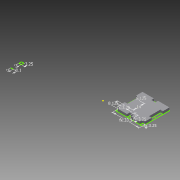
# Autodesk Inventor part: arm-servo
Saved by Autodesk Inventor 2013 (Build 170138000, 138)
## iProperties
Created: 2012-09-08
Part Number: arm-servo
Material: Generic
Document SubType Name: Modeling
Designer: frankenteddy
Density: 1 g/cm^3
Author: frankenteddy
Autodesk Inventor part; units mm, degrees
ref_plane "YZ Plane" through (0, 0, 0) normal (1, 0, 0) x (0, 1, 0)
ref_plane "XZ Plane" through (0, 0, 0) normal (0, 1, 0) x (-1, 0, 0)
ref_plane "XY Plane" through (0, 0, 0) normal (0, 0, 1) x (1, 0, 0)
sketch "Block1" plane through (0, 0, 0) normal (0, 0, 1) x (1, 0, 0)
  circle A0 centre (74.029, 24.2723) radius 1
  line L0 (49.279, 30.4723) -> (71.779, 30.4723)
  line L1 (71.779, 30.4723) -> (71.779, 18.0723)
  line L2 (71.779, 18.0723) -> (49.279, 18.0723)
  line L3 (49.279, 18.0723) -> (49.279, 30.4723)
  line L4 (49.279, 30.4723) -> (44.779, 30.4723)
  line L5 (44.779, 30.4723) -> (44.779, 18.0723)
  line L6 (44.779, 18.0723) -> (49.279, 18.0723)
  line L7 (49.279, 18.0723) -> (49.279, 30.4723)
  line L8 (71.779, 30.4723) -> (76.279, 30.4723)
  line L9 (76.279, 30.4723) -> (76.279, 18.0723)
  line L10 (76.279, 18.0723) -> (71.779, 18.0723)
  line L11 (71.779, 18.0723) -> (71.779, 30.4723)
  line L12 (44.779, 24.2723) -> (76.279, 24.2723) construction
  line L13 (47.029, 30.4723) -> (47.029, 18.0723) construction
  circle A1 centre (47.029, 24.2723) radius 1
  line L14 (74.029, 30.4723) -> (74.029, 18.0723) construction
  point P0 (60.979, 24.0984)
  dimension "d7" = 22.5
  dimension "d8" = 12.4
  dimension "d9" = 4.5
  dimension "d10" = 4.5
  dimension "d11" = 2
  dimension "d12" = 2
  measures "d7" distance of L1.end L2.end
  measures "d8" distance of L0.end L1.end
  measures "d9" distance of L6.end L5.end
  measures "d10" distance of L9.end L10.end
  measures "d11" diameter of A0
  measures "d12" diameter of A1
sketch "Sketch1" plane through (0, 0, 0) normal (0, 0, 1) x (1, 0, 0)
  line L0 (-92.7646, -8.503) -> (-89.7646, -8.503)
  line L1 (-89.7646, -8.503) -> (-89.7646, -11.753)
  line L2 (-89.7646, -11.753) -> (-92.7646, -11.753)
  line L3 (-92.7646, -11.753) -> (-92.7646, -8.503)
  line L4 (-92.7646, -21.6527) -> (-89.7646, -21.6527)
  line L5 (-89.7646, -21.6527) -> (-89.7646, -21.7527)
  line L6 (-89.7646, -21.7527) -> (-92.7646, -21.7527)
  line L7 (-92.7646, -21.7527) -> (-92.7646, -21.6527)
  line L8 (18.2857, 30.9706) -> (51.7857, 30.9706)
  line L9 (51.7857, 30.9706) -> (51.7857, 0.7206)
  line L10 (51.7857, 0.7206) -> (18.2857, 0.7206)
  line L11 (18.2857, 0.7206) -> (18.2857, 30.9706)
  line L12 (18.2857, 22.8456) -> (21.5357, 22.8456)
  line L13 (21.5357, 22.8456) -> (21.5357, 8.8456)
  line L14 (21.5357, 8.8456) -> (18.2857, 8.8456)
  line L15 (18.2857, 8.8456) -> (18.2857, 22.8456)
  line L16 (35.0357, 30.9706) -> (35.0357, 0.7206) construction
  line L17 (51.7857, 22.8456) -> (48.5357, 22.8456)
  line L18 (48.5357, 22.8456) -> (48.5357, 8.8456)
  line L19 (48.5357, 8.8456) -> (51.7857, 8.8456)
  line L20 (51.7857, 8.8456) -> (51.7857, 22.8456)
  line L21 (32.5357, -2.5294) -> (37.5357, -2.5294)
  line L22 (37.5357, -2.5294) -> (37.5357, 0.7206)
  line L23 (37.5357, 0.7206) -> (32.5357, 0.7206)
  line L24 (32.5357, 0.7206) -> (32.5357, -2.5294)
  line L25 (35.0357, 0.7206) -> (35.0357, -2.5294) construction
  line L26 (18.2857, 14.2206) -> (51.7857, 14.2206) construction
  line L27 (32.5357, 30.9706) -> (37.5357, 30.9706)
  line L28 (37.5357, 30.9706) -> (37.5357, 27.7206)
  line L29 (37.5357, 27.7206) -> (32.5357, 27.7206)
  line L30 (32.5357, 27.7206) -> (32.5357, 30.9706)
  line L31 (35.0357, 27.7206) -> (35.0357, 30.9706) construction
  line L32 (18.2857, 0.7206) -> (51.7857, 0.7206)
  line L33 (51.7857, 0.7206) -> (51.7857, -2.5294)
  line L34 (51.7857, -2.5294) -> (18.2857, -2.5294)
  line L35 (18.2857, -2.5294) -> (18.2857, 0.7206)
  line L36 (18.2857, -2.5294) -> (21.5357, -2.5294)
  line L37 (21.5357, -2.5294) -> (21.5357, 0.7206)
  line L38 (21.5357, 0.7206) -> (18.2857, 0.7206)
  line L39 (18.2857, 0.7206) -> (18.2857, -2.5294)
  line L40 (51.7857, -2.5294) -> (48.5357, -2.5294)
  line L41 (48.5357, -2.5294) -> (48.5357, 0.7206)
  line L42 (48.5357, 0.7206) -> (51.7857, 0.7206)
  line L43 (51.7857, 0.7206) -> (51.7857, -2.5294)
  point P0 (0, 0)
  point P1 (35.0357, 27.7206)
  dimension "d0" = 3
  dimension "mat" = 3.25
  dimension "d2" = 3
  dimension "d3" = 0.1
  dimension "d32" = 33.5
  dimension "d34" = 3.25
  dimension "d35" = 14
  dimension "d36" = 8.125
  dimension "d39" = 5
  dimension "d40" = 3.25
  dimension "d45" = 8.125
  dimension "d46" = 3.25
  constraints: 88 end point, 16 parallel, 11 symmetric about line, 9 perpendicular, 8 horizontal, 4 collinear, 4 midpoint, 4 point on line
  measures "d0" distance of L1.end L3.start
  measures "mat" distance of L1.start L1.end
  measures "d2" distance of L5.end L7.start
  measures "d3" distance of L5.start L5.end
  measures "d32" distance of L9.end L10.end
  measures "d34" distance of L13.end L14.end
  measures "d35" distance of L12.end L13.end
  measures "d36" distance between parallel lines of L12 L8
  measures "d39" distance of L23.end L22.end
  measures "d40" distance of L22.end L21.end
  measures "d45" distance between parallel lines of L10 L14
  measures "d46" distance of L32.end L33.end
extrude "Extrusion3" add sketch "Sketch1" along normal blind 3.25 contours L8 L30 L29 L28 L9 L17 L18 L19 L10 L11 L14 L13 L12 | L8 L28 L29 L30
extrude "Extrusion6" add sketch "Sketch1" along normal blind 3.25 contours L10 L37 L34 L35 | L10 L24 L34 L37 | L33 L34 L41 L10 | L10 L41 L34 L22
extrude "Extrusion7" cut sketch "Sketch1" along normal blind 3.25 contours L10 L37 L34 L35 | L33 L34 L41 L10
extrude "Extrusion8" cut sketch "Sketch1" along normal blind 3.25 contours L8 L28 L29 L30
equation "\"d34\" = mat"
equation "\"d40\" = mat"
equation "\"d46\" = mat"
equation "\"d37\" = mat"
equation "\"d47\" = mat"
equation "\"d49\" = mat"
equation "\"d51\" = mat"
body "Solid3"
